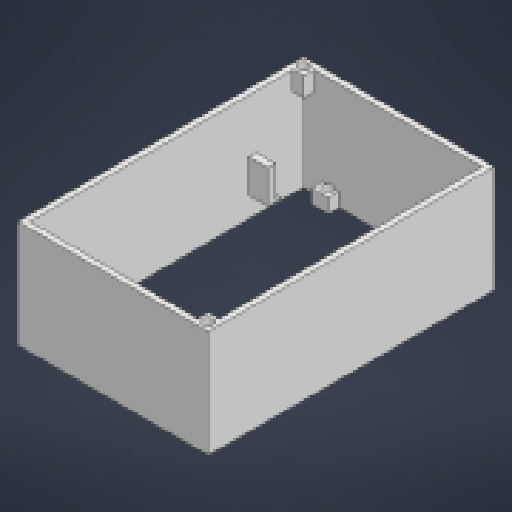
# Autodesk Inventor part: PCB_Housing_03_V4
Saved by Autodesk Inventor 2026.2 (Build 302298000, 298)
## iProperties
Created: 2026-03-15
Part Number: PCB_Housing_03_V4
Material: Generic
Document SubType Name: Modeling
Designer: vckot
Density: 1 g/cm^3
Appearance: Default
Author: vckot
Autodesk Inventor part; units mm, degrees
ref_plane "YZ Plane" through (0, 0, 0) normal (1, 0, 0) x (0, 1, 0)
ref_plane "XZ Plane" through (0, 0, 0) normal (0, 1, 0) x (-1, 0, 0)
ref_plane "XY Plane" through (0, 0, 0) normal (0, 0, 1) x (1, 0, 0)
sketch "Sketch2" plane through (0, 0, 0) normal (0, 1, 0) x (1, 0, 0)
  line L0 (40, -60) -> (40, 60)
  line L1 (40, 60) -> (-40, 60)
  line L2 (-40, 60) -> (-40, -60)
  line L3 (-40, -60) -> (40, -60)
  line L4 (-37.5, -57.5) -> (-37.5, 57.5)
  line L5 (-37.5, 57.5) -> (37.5, 57.5)
  line L6 (37.5, 57.5) -> (37.5, -57.5)
  line L7 (37.5, -57.5) -> (-37.5, -57.5)
  line L8 (32.5, -37.5) -> (37.5, -37.5)
  line L9 (32.5, -37.5) -> (32.5, -40)
  line L10 (32.5, -40) -> (37.5, -40)
  point P0 (0, 0)
  point P1 (40, 0)
  point P2 (0, 60)
  point P3 (0, 0)
  dimension "d4" = 2.5
  dimension "d7" = 120
  dimension "d8" = 80
  dimension "d9" = 20
  dimension "d10" = 5
  dimension "d11" = 2.5
  constraints: 22 end point, 4 perpendicular, 2 midpoint, 2 point on line, 1 coincident, 1 horizontal, 1 horizontal alignment, 1 vertical, 1 vertical alignment, 3 other
  measures "d4" distance between parallel lines of L2 L4
  measures "d7" distance of L0.start L0.end
  measures "d8" distance of L0.end L1.end
  measures "d9" distance between parallel lines of L7 L8
  measures "d10" distance of L8.start L8.end
  measures "d11" distance of L8.start L9.end
extrude "Extrusion2" add sketch "Sketch2" along normal blind 45
extrude "Extrusion3" add sketch "Sketch2" along normal blind 2.5 contours L10 L9 L8 L6
sketch "Sketch3" plane through (-37.5, 0, 57.5) normal (1, 0, 0) x (0, 0, -1)
  line L0 (95.08, 8.5) -> (95.08, 22.5)
  line L1 (115, 0) -> (115, 45) projected
  line L2 (95.08, 8.5) -> (92.08, 8.5)
  line L3 (92.08, 8.5) -> (92.08, 22.5)
  line L4 (117.5, 0) -> (-2.5, 0) projected
  line L5 (95.08, 22.5) -> (92.08, 22.5)
  point P0 (57.5, 0)
  dimension "d14" = 19.92
  dimension "d15" = 3
  dimension "d16" = 8.5
  dimension "d17" = 14
  constraints: 8 end point, 2 horizontal, 1 perpendicular, 1 vertical
  measures "d14" distance between parallel lines of L1 L0
  measures "d15" distance between parallel lines of L0 L3
  measures "d16" distance between parallel lines of L4 L2
  measures "d17" distance between parallel lines of L2 L5
extrude "Extrusion4" add sketch "Sketch3" along normal blind 8
sketch "Sketch4" plane through (-37.5, 8.5, -37.58) normal (0, 0, -1) x (-1, 0, 0)
  line L0 (-8, 0) -> (-8, 14) projected
  line L1 (-8, 0) -> (0, 0)
  line L2 (0, 0) -> (0, 1)
  line L3 (0, 1) -> (-8, 1)
  line L4 (-8, 1) -> (-8, 0)
  line L5 (0, 14) -> (0, 0) projected
  line L6 (0, 0) -> (-8, 0) projected
  point P0 (-37.5, -8.5)
  point P1 (-8, 1)
  dimension "d20" = 1
  constraints: 8 end point, 2 parallel, 1 collinear, 1 horizontal, 1 perpendicular
  measures "d20" distance between parallel lines of L6 L3
extrude "Extrusion5" add sketch "Sketch4" along normal blind 2
sketch "Sketch5" plane through (0, 0, 0) normal (0, -1, 0) x (1, 0, 0)
  line L0 (-40, 60) -> (40, 60) projected
  line L1 (-40, 60) -> (-33, 60)
  line L2 (-33, 60) -> (-33, 53)
  line L3 (-33, 53) -> (-40, 53)
  line L4 (-40, 53) -> (-40, 60)
  line L5 (40, 60) -> (40, -60) projected
  line L6 (40, 60) -> (33, 60)
  line L7 (33, 60) -> (33, 53)
  line L8 (33, 53) -> (40, 53)
  line L9 (40, 53) -> (40, 60)
  line L10 (40, -60) -> (-40, -60) projected
  line L11 (-29.5, -60) -> (-22.5, -60)
  line L12 (-22.5, -60) -> (-22.5, -53)
  line L13 (-22.5, -53) -> (-29.5, -53)
  line L14 (-29.5, -53) -> (-29.5, -60)
  line L15 (-29.5, -34.58) -> (-29.5, -39.58) projected
  point P0 (0, 0)
  dimension "d23" = 7
  dimension "d24" = 7
  dimension "d25" = 7
  dimension "d26" = 7
  dimension "d27" = 7
  dimension "d28" = 7
  dimension "d29" = 0
  constraints: 24 end point, 6 parallel, 3 horizontal, 3 perpendicular, 1 point on line
  measures "d23" distance of L2.end L3.end
  measures "d24" distance of L1.end L2.end
  measures "d25" distance of L8.end L7.end
  measures "d26" distance of L7.end L6.end
  measures "d27" distance of L13.end L12.end
  measures "d28" distance of L12.end L11.end
  measures "d29" distance between parallel lines of L15 L14
extrude "Extrusion6" add sketch "Sketch5" against normal blind 6
sketch "Sketch6" plane through (0, 0, 0) normal (0, -1, 0) x (1, 0, 0)
  line L0 (-37.5, 53) -> (-33, 53) projected
  line L1 (-33, 53) -> (-33, 57.5) projected
  line L2 (33, 53) -> (37.5, 53) projected
  line L3 (33, 57.5) -> (33, 53) projected
  line L4 (40, -60) -> (-40, -60) projected
  line L5 (-22.5, -57.5) -> (-22.5, -53) projected
  point P0 (0, 0)
  point P1 (-26, -56.5)
  point P2 (-36.5, 56.5)
  point P3 (36.5, 56.5)
  point P4 (35.25, 53)
  dimension "d32" = 3.5
  dimension "d33" = 3.5
  dimension "d34" = 3.5
  dimension "d35" = 3.5
  dimension "d36" = 3.5
  dimension "d37" = 3.5
  constraints: 1 midpoint
  measures "d32" distance from line of L0 point (-36.5, 56.5)
  measures "d33" distance from line of L1 point (-36.5, 56.5)
  measures "d34" vertical distance of point (35.25, 53) point (36.5, 56.5)
  measures "d35" distance from line of L3 point (36.5, 56.5)
  measures "d36" distance from line of L4 point (-26, -56.5)
  measures "d37" distance from line of L5 point (-26, -56.5)
hole "Hole1" at (-26, 0, -56.5) at (-36.5, 0, 56.5) at (36.5, 0, 56.5) direction (0, 1, 0) diameter 4.5 depth 6 tip angle 118
sketch "Sketch7" plane through (0, 45, 0) normal (0, 1, 0) x (1, 0, 0)
  line L0 (-40, 60) -> (-40, -60) projected
  line L1 (-40, 60) -> (-33, 60)
  line L2 (-33, 60) -> (-33, 53)
  line L3 (-33, 53) -> (-40, 53)
  line L4 (-40, 53) -> (-40, 60)
  line L5 (-40, -60) -> (40, -60) projected
  line L6 (40, -60) -> (33, -60)
  line L7 (33, -60) -> (33, -53)
  line L8 (33, -53) -> (40, -53)
  line L9 (40, -53) -> (40, -60)
  circle A0 centre (36.5, -56.5) radius 2.25 projected
  point P0 (0, 0)
  point P1 (-36.5, 56.5)
  point P2 (-33, 56.5)
  point P3 (-36.5, 53)
  dimension "d45" = 7
  dimension "d46" = 7
  dimension "d47" = 7
  dimension "d48" = 7
  constraints: 16 end point, 4 parallel, 2 horizontal, 2 midpoint, 2 perpendicular, 1 coincident, 1 horizontal alignment, 1 vertical alignment
  measures "d45" distance of L2.end L3.end
  measures "d46" distance of L1.end L2.end
  measures "d47" distance of L7.end L8.end
  measures "d48" distance of L6.end L7.end
extrude "Extrusion7" add sketch "Sketch7" against normal blind 8 contours L1 L2 L3 L0 | L7 L8 L9 L5 | A0
hole "Hole2" at (36.5, 45, 56.5) at (-36.5, 45, -56.5) direction (0, -1, 0) diameter 4.5 depth 8 tip angle 118
body "Solid1"
